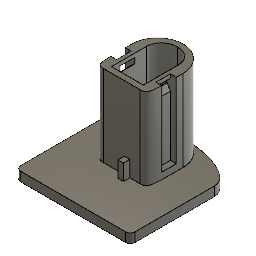
battery_shore_plug (Autodesk Fusion 360 design; units mm, degrees)
Autodesk Fusion 360 part; units mm, degrees
sketch "MountingFace" plane through (0, 0, 0) normal (0, 1, 0) x (1, 0, 0) in component "Battery"
  line L0 (-28.11, 0) -> (0, 0)
  line L1 (-30.65, 2.54) -> (-30.65, 45)
  arc A0 (-30.65, 2.54) -> (-28.11, 0) centre (-28.11, 2.54) ccw
  line L2 (-30.65, 45) -> (-30.65, 53)
  line L3 (-30.65, 53) -> (-15, 58.8)
  line L4 (-15, 58.8) -> (0, 58.8)
  spline S0 degree 3 poles (-30.65, 45) (-30.65, 53) (-15, 58.8) (0, 58.8) knots 0 0 0 0 1 1 1 1
  line L5 (0, 58.8) -> (20, 58.8) construction
  line L6 (0, 0) -> (0, 70) construction
  spline S1 degree 3 poles (30.65, 45) (30.65, 53) (15, 58.8) (0, 58.8) knots 0 0 0 0 1 1 1 1
  line L7 (30.65, 45) -> (30.65, 53)
  line L8 (30.65, 53) -> (15, 58.8)
  line L9 (15, 58.8) -> (0, 58.8)
  line L10 (30.65, 2.54) -> (30.65, 45)
  line L11 (28.11, 0) -> (0, 0)
  arc A1 (28.11, 0) -> (30.65, 2.54) centre (28.11, 2.54) ccw
  dimension "d1" = 2.54
  dimension "d2" = 20
  dimension "d3" = 61.3
  dimension "d4" = 58.8
  dimension "d5" = 45
  dimension "d6" = 8
  dimension "d7" = 15
  measures "d1" radius of A0
  measures "d3" distance of L1 L10
  measures "d7" distance of L0.end
extrude "Extrude1" add sketch "MountingFace" against normal blind 5 contours L0 L1 A0 S0 S1 L10 L11 A1 in component "Battery"
sketch "TerminalPost" plane through (0, 0, 0) normal (0, 1, 0) x (-1, 0, 0) in component "Battery"
  arc A0 (30.65, -2.54) -> (28.11, 0) centre (28.11, -2.54) ccw
  line L0 (28.11, 0) -> (-28.11, 0)
  arc A1 (-28.11, 0) -> (-30.65, -2.54) centre (-28.11, -2.54) ccw
  line L1 (-30.65, -2.54) -> (-30.65, -45)
  spline S0 degree 3 poles (-30.65, -45) (-30.65, -53) (-15, -58.8) (0, -58.8) knots 0 0 0 0 1 1 1 1
  spline S1 degree 3 poles (30.65, -45) (30.65, -53) (15, -58.8) (0, -58.8) knots 0 0 0 0 1 1 1 1
  line L2 (30.65, -45) -> (30.65, -2.54)
  spline S2 degree 3 poles (30.65, -45) (30.65, -53) (15, -58.8) (0, -58.8) knots 0 0 0 0 1 1 1 1
  arc A2 (0, -58.8) -> (13.7, -45.1) centre (0, -45.1) ccw
  line L3 (13.7, -45.1) -> (13.6945, -27.1)
  line L4 (13.6945, -27.1) -> (13.75, -26.1)
  line L5 (13.75, -26.1) -> (9.75, -26.1)
  spline S3 degree 3 poles (13.7, -45.1) (13.6945, -27.1) (13.75, -26.1) (9.75, -26.1) knots 0 0 0 0 1 1 1 1
  line L6 (9.75, -26.1) -> (0, -26.1)
  line L7 (0, 0) -> (0, -26.1) construction
  line L8 (0, -26.1) -> (0, -58.8) construction
  line L9 (-9.75, -26.1) -> (0, -26.1)
  spline S4 degree 3 poles (-13.7, -45.1) (-13.6945, -27.1) (-13.75, -26.1) (-9.75, -26.1) knots 0 0 0 0 1 1 1 1
  line L10 (-13.7, -45.1) -> (-13.6945, -27.1)
  line L11 (-13.6945, -27.1) -> (-13.75, -26.1)
  line L12 (-13.75, -26.1) -> (-9.75, -26.1)
  arc A3 (-13.7, -45.1) -> (0, -58.8) centre (0, -45.1) ccw
  dimension "d10" = 32.7
  dimension "d11" = 27.4
  dimension "d12" = 19.5
  dimension "d13" = 18
  dimension "d14" = 4
  dimension "d68" = 1
  measures "d10" distance of L7.start
extrude "Extrude2" add sketch "TerminalPost" along normal blind 43.5 contours A2 S3 L6 L9 S4 A3 in component "Battery"
sketch "TerminalCutout" plane through (0, 43.5, 0) normal (0, 1, 0) x (-1, 0, 0) in component "Battery"
  spline S0 degree 3 poles (-9.75, -26.1) (-13.75, -26.1) (-13.6945, -27.1) (-13.7, -45.1) knots -1 -1 -1 -1 0 0 0 0
  arc A0 (-13.7, -45.1) -> (13.7, -45.1) centre (0, -45.1) ccw construction
  spline S1 degree 3 poles (13.7, -45.1) (13.6945, -27.1) (13.75, -26.1) (9.75, -26.1) knots 0 0 0 0 1 1 1 1 construction
  line L0 (9.75, -26.1) -> (-9.75, -26.1)
  spline S2 degree 3 poles (13.7, -45.1) (13.6945, -27.1) (13.75, -26.1) (9.75, -26.1) knots 0 0 0 0 1 1 1 1
  arc A1 (-13.7, -45.1) -> (13.7, -45.1) centre (0, -45.1) ccw
  line L1 (16.55, -41.5) -> (10.55, -41.5)
  line L2 (10.55, -41.5) -> (10.55, -33.8)
  line L3 (10.55, -33.8) -> (16.55, -33.8)
  line L4 (16.55, -33.8) -> (16.55, -41.5)
  line L5 (0, -45.1) -> (0, -24.3) construction
  line L6 (-10.55, -41.5) -> (-10.55, -33.8)
  line L7 (-16.55, -41.5) -> (-10.55, -41.5)
  line L8 (-16.55, -33.8) -> (-16.55, -41.5)
  line L9 (-10.55, -33.8) -> (-16.55, -33.8)
  dimension "d29" = 21.1
  dimension "d30" = 7.7
  dimension "d31" = 7.7
  dimension "d32" = 6
extrude "Extrude4" cut sketch "TerminalCutout" against normal blind 40 contours S0 L6 L7 L9 | S0 L7 L8 L9 | S2 L1 L3 L4 | S2 L1 L2 L3 in component "Battery"
sketch "TopAlignmentPin" plane through (0, 0, 0) normal (0, 1, 0) x (-1, 0, 0) in component "Battery"
  arc A0 (30.65, -2.54) -> (28.11, 0) centre (28.11, -2.54) ccw
  line L0 (28.11, 0) -> (-28.11, 0)
  arc A1 (-28.11, 0) -> (-30.65, -2.54) centre (-28.11, -2.54) ccw
  line L1 (-30.65, -2.54) -> (-30.65, -45)
  spline S0 degree 3 poles (-30.65, -45) (-30.65, -53) (-15, -58.8) (0, -58.8) knots 0 0 0 0 1 1 1 1
  arc A2 (-13.7, -45.1) -> (0, -58.8) centre (0, -45.1) ccw
  spline S1 degree 3 poles (-13.7, -45.1) (-13.6945, -27.1) (-13.75, -26.1) (-9.75, -26.1) knots 0 0 0 0 1 1 1 1
  line L2 (-9.75, -26.1) -> (9.75, -26.1) construction
  spline S2 degree 3 poles (9.75, -26.1) (13.75, -26.1) (13.6945, -27.1) (13.7, -45.1) knots -1 -1 -1 -1 0 0 0 0
  arc A3 (0, -58.8) -> (13.7, -45.1) centre (0, -45.1) ccw
  spline S3 degree 3 poles (30.65, -45) (30.65, -53) (15, -58.8) (0, -58.8) knots 0 0 0 0 1 1 1 1
  line L3 (30.65, -45) -> (30.65, -2.54)
  line L4 (0, 0) -> (0, -38) construction
  line L5 (-1.3, -26.1) -> (-4.3, -26.1)
  line L6 (-4.3, -26.1) -> (-4.3, -22.7)
  line L7 (-4.3, -22.7) -> (-1.3, -22.7)
  line L8 (-1.3, -22.7) -> (-1.3, -26.1)
  dimension "d47" = 3
  dimension "d48" = 3.4
  dimension "d49" = 4.3
extrude "Extrude7" add sketch "TopAlignmentPin" along normal blind 8.5 contours L5 L6 L7 L8 in component "Battery"
sketch "Central Cavity" plane through (0, 43.5, 0) normal (0, 1, 0) x (-1, 0, 0) in component "Battery"
  line L0 (13.6983, -41.5) -> (10.55, -41.5)
  line L1 (10.55, -41.5) -> (10.55, -33.8)
  line L2 (10.55, -33.8) -> (13.6244, -33.8)
  spline S0 degree 3 poles (13.6244, -33.8) (13.4202, -26.6269) (12.6535, -26.1) (9.75, -26.1) knots 0.274126 0.274126 0.274126 0.274126 1 1 1 1
  line L3 (9.75, -26.1) -> (-9.75, -26.1)
  spline S1 degree 3 poles (-9.75, -26.1) (-12.6535, -26.1) (-13.4202, -26.6269) (-13.6244, -33.8) knots -1 -1 -1 -1 -0.274126 -0.274126 -0.274126 -0.274126
  line L4 (-13.6244, -33.8) -> (-10.55, -33.8)
  line L5 (-10.55, -33.8) -> (-10.55, -41.5)
  line L6 (-10.55, -41.5) -> (-13.6983, -41.5)
  spline S2 degree 3 poles (-13.6983, -41.5) (-13.6995, -42.6173) (-13.6996, -43.8153) (-13.7, -45.1) knots -0.07137 -0.07137 -0.07137 -0.07137 0 0 0 0
  arc A0 (-13.7, -45.1) -> (13.7, -45.1) centre (0, -45.1) ccw
  spline S3 degree 3 poles (13.7, -45.1) (13.6996, -43.8153) (13.6995, -42.6173) (13.6983, -41.5) knots 0 0 0 0 0.07137 0.07137 0.07137 0.07137
  line L7 (0, -29.1) -> (-8.55, -29.1)
  line L8 (-8.55, -29.1) -> (-8.55, -47.8189)
  line L9 (0, 0) -> (0, -105) construction
  arc A1 (-8.55, -47.8189) -> (0, -55.8) centre (-0.55, -47.8189) ccw
  arc A2 (0, -55.8) -> (8.55, -47.8189) centre (0.55, -47.8189) ccw
  line L10 (8.55, -29.1) -> (8.55, -47.8189)
  line L11 (0, -29.1) -> (8.55, -29.1)
  line L12 (9.75, -26.1) -> (-9.75, -26.1)
  arc A3 (-13.7, -45.1) -> (13.7, -45.1) centre (0, -45.1) ccw
  line L13 (-10.55, -33.8) -> (-10.55, -41.5)
  line L14 (-10.55, -41.5) -> (-8.55, -41.5) construction
  line L15 (0, -55.8) -> (0, -58.8) construction
  line L16 (0, -29.1) -> (0, -26.1) construction
  dimension "d70" = 8
  dimension "d71" = 2
  dimension "d72" = 3
  measures "d70" radius of A1
  measures "d72" distance of L9.start
sketch "Terminal Insertion Hole" plane through (10.55, 0, 0) normal (1, 0, 0) x (0, 0, -1) in component "Battery"
  line L0 (41.5, 43.5) -> (33.8, 43.5)
  line L1 (33.8, 43.5) -> (33.8, 3.5)
  line L2 (33.8, 3.5) -> (41.5, 3.5)
  line L3 (41.5, 3.5) -> (41.5, 43.5)
  line L4 (33.8, 43.5) -> (41.5, 43.5)
  line L5 (33.8, 41.5) -> (41.5, 41.5)
  line L6 (41.5, 41.5) -> (41.5, 43.5) construction
  line L7 (33.8, 41.5) -> (33.8, 38.5)
  line L8 (33.8, 38.5) -> (41.5, 38.5)
  dimension "d75" = 3
  dimension "d81" = 5
extrude "Extrude12" cut sketch "Central Cavity" against normal through all contours L7 L8 A1 A2 L10 L11 in component "Battery"
extrude "Extrude13" cut sketch "Terminal Insertion Hole" against normal through all contours L1 L3 L5 L7 L8 in component "Battery"
chamfer "Chamfer2" distance 3 angle 30 2 edges at (-10.55, 38.5, -37.65) (10.55, 38.5, -37.65) measured on face at (-10.55, 26.8333, -38.9333) measured on face at (10.55, 26.8333, -38.9333) in component "Battery"
component "Battery" placed x (1, 0, 0) y (0, 1, 0) z (0, 0, 1) at (0, 0, 0)
